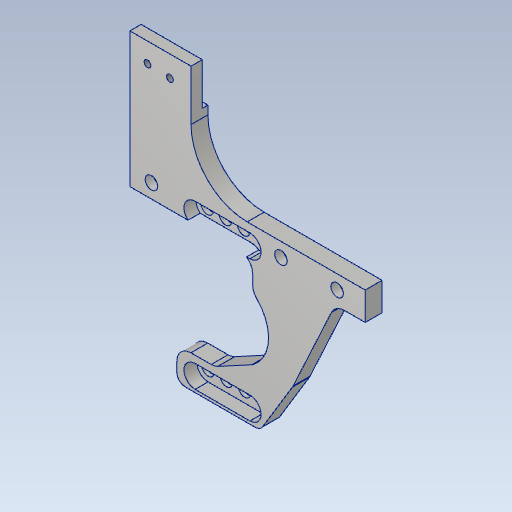
# Autodesk Inventor part: Extruder bracket
Saved by Autodesk Inventor 2020 (Build 240168000, 168)
## iProperties
Created: 2018-10-20
Part Number: Extruder bracket
Material: Aluminum 6061
Document SubType Name: Modeling
Designer: LillaHunden
Density: 2.7 g/cm^3
Appearance: Aluminum - Flat
Mass: 27.8066 g
Surface Area: 65.7368 cm^2
Volume: 10.2987 cm^3
Author: LillaHunden
Autodesk Inventor part; units mm, degrees
sketch "Sketch3" plane through (0, 0, 0) normal (0, 0, 1) x (1, 0, 0)
  line L0 (-29.642335, -32.061774) -> (11.628959, -32.061774)
  line L1 (11.628959, -32.061774) -> (11.628959, 19.831605)
  line L2 (11.628959, 19.831605) -> (37.40227, 19.831605)
  line L3 (37.40227, 19.831605) -> (37.40227, 29.831605)
  line L4 (37.40227, 29.831605) -> (-52.692966, 29.831605)
  line L5 (-52.692966, 29.831605) -> (-52.692966, 19.831605)
  line L6 (-52.692966, 19.831605) -> (-2.658885, 19.831605)
  line L7 (-2.658885, 19.831605) -> (-2.658885, -20.52891)
  line L8 (-2.658885, -20.52891) -> (-29.642335, -20.52891)
  line L9 (-29.642335, -20.52891) -> (-29.642335, -32.061774)
  line L10 (37.40227, 19.831605) -> (-46.39773, 19.831605)
  point P0 (0, 0)
  constraints: 20 end point, 9 perpendicular, 1 horizontal, 1 horizontal alignment, 1 point on line
extrude "Extrusion3" add sketch "Sketch3" along normal blind 6
sketch "Sketch4" plane through (0, 0, 6) normal (0, 0, 1) x (1, 0, 0)
  circle A0 centre (-10.748341, -2.098696) radius 3.15 construction
  circle A1 centre (-10.748341, -2.098696) radius 13.750611
  point P0 (0, 0)
  constraints: 1 centre point, 1 coincident
extrude "Extrusion4" cut sketch "Sketch4" against normal through all
sketch "Sketch5" plane through (0, 0, 0) normal (0, 0, -1) x (-1, 0, 0)
  line L0 (-11.628959, -32.061774) -> (-11.628959, 19.831605)
  line L1 (-11.628959, -12.820332) -> (-26.727339, 19.831605)
  line L2 (-11.628959, 19.831605) -> (-37.40227, 19.831605)
  point P0 (0, 0)
  constraints: 2 end point, 2 point on line
extrude "Extrusion5" add sketch "Sketch5" against normal up to surface (6 mm away)
sketch "Sketch6" plane through (0, 0, 6) normal (0, 0, 1) x (1, 0, 0)
  line L0 (-2.658885, -20.52891) -> (-29.642335, -20.52891)
  line L1 (-2.658885, -13.21805) -> (-2.658885, -20.52891)
  line L2 (-16.15061, -20.52891) -> (-2.658885, -13.21805)
  point P0 (0, 0)
  constraints: 2 end point, 2 midpoint
ref_plane "Work Plane1" through (-29.642335, -32.061774, 0) normal (0, 0, 1) x (1, 0, 0)
extrude "Extrusion6" add sketch "Sketch6" against normal up to surface (6 mm away)
sketch "Sketch7" plane through (0, 0, 0) normal (0, 0, -1) x (-1, 0, 0)
  line L0 (29.642335, -32.061774) -> (-11.628959, -32.061774)
  line L1 (0, -32.061774) -> (-11.628959, -12.820332)
  line L2 (-11.628959, -32.061774) -> (-11.628959, -12.820332)
  point P0 (0, 0)
  constraints: 2 end point, 1 point on line
extrude "Extrusion7" cut sketch "Sketch7" against normal through all
fillet "Fillet1" radius 5 6 edges at (-16.1506, -20.5289, 3) (-2.6589, -13.218, 3) (11.629, -12.8203, 3) (26.7273, 19.8316, 3) (-2.6589, 9.0207, 3) (-2.6589, 19.8316, 3)
fillet "Fillet2" radius 3 1 edges at (-29.6423, -32.0618, 3)
fillet "Fillet3" radius 3 1 edges at (0, -32.0618, 3)
sketch "Sketch8" plane through (0, 0, 0) normal (0, 0, -1) x (-1, 0, 0)
  line L0 (52.59773, 19.831605) -> (-37.40227, 19.831605) construction
  line L1 (-37.40227, 19.831605) -> (-37.40227, 29.831605) construction
  line L2 (52.59773, 29.831605) -> (-37.40227, 29.831605) construction
  line L3 (52.59773, 19.831605) -> (52.59773, 29.831605) construction
  line L4 (-37.40227, 19.831605) -> (-37.40227, 29.831605) construction
  line L5 (-37.40227, 24.831605) -> (52.692966, 24.831605) construction
  line L6 (52.692966, 29.831605) -> (52.692966, 19.831605) construction
  point P0 (0, 0)
  point P1 (-27.40227, 24.831605)
  point P2 (-7.40227, 24.831605)
  point P3 (38.692966, 24.831605)
  dimension "d20" = 10
  dimension "d21" = 14
  dimension "d23" = 20
  constraints: 3 point on line, 2 end point, 2 midpoint
  measures "d20" distance from line of L1 point (-27.402, 24.832)
  measures "d21" distance from line of L6 point (38.693, 24.832)
  measures "d23" distance of point (-7.402, 24.832) point (-27.402, 24.832)
sketch "Sketch9" plane through (0, 0, 0) normal (0, 0, -1) x (-1, 0, 0)
  point P0 (-27.40227, 24.831605)
  point P1 (-7.40227, 24.831605)
  point P2 (38.692966, 24.831605)
hole "Hole1" at (27.40227, 24.831605, 0) at (7.40227, 24.831605, 0) at (-38.692966, 24.831605, 0) direction (0, 0, 1) diameter 4.5 depth 6 counterbore diameter 8.1 counterbore depth 3
sketch "Sketch11" plane through (0, 0, 0) normal (0, 0, -1) x (-1, 0, 0)
  arc A0 (1.642335, 27.938226) -> (-1.357665, 24.938226) centre (1.642335, 24.938226) ccw construction
  line L0 (-1.357665, 12.938226) -> (-1.357665, 24.938226) construction
  line L1 (-1.357665, 12.938226) -> (29.642335, 12.938226) construction
  line L2 (29.642335, 24.938226) -> (29.642335, 12.938226) construction
  arc A1 (29.642335, 24.938226) -> (26.642335, 27.938226) centre (26.642335, 24.938226) ccw construction
  line L3 (1.642335, 27.938226) -> (26.642335, 27.938226) construction
  circle A2 centre (10.142335, 22.938226) radius 2.15
  circle A3 centre (23.142335, 22.938226) radius 2.15
  circle A4 centre (16.642335, 22.938226) radius 2.15
  circle A5 centre (3.642335, 22.938226) radius 2.15
  point P0 (0, 0)
  point P1 (16.642335, 22.938226)
  point P2 (10.142335, 22.938226)
  point P3 (3.642335, 22.938226)
sketch "Sketch12" plane through (0, 0, 6) normal (0, 0, 1) x (1, 0, 0)
  point P0 (-3.642335, -27.061774)
  point P1 (-23.142335, -27.061774)
  point P2 (-16.642335, -27.061774)
  point P3 (-10.142335, -27.061774)
hole "Hole5" at (-3.642335, -27.061774, 6) at (-23.142335, -27.061774, 6) at (-16.642335, -27.061774, 6) at (-10.142335, -27.061774, 6) direction (0, 0, -1) diameter 4.5 depth 6 counterbore diameter 8 counterbore depth 4.6
sketch "Sketch13" plane through (-52.692966, 19.831605, 0) normal (-1, 0, 0) x (0, 0, 1)
  line L0 (0, 10) -> (0, 0) projected
  line L1 (0, 0) -> (6, 0) projected
  line L2 (6, 10) -> (6, 0) projected
  line L3 (0, 10) -> (6, 10) projected
  point P0 (0, -19.831605)
ref_plane "Work Plane2" through (-46.59773, 19.831605, 6) normal (-1, 0, 0) x (0, 0, 1)
extrude "Extrusion8" cut sketch "Sketch13" against normal up to surface (6.095236 mm away)
chamfer "Chamfer2" distance 0.1 angle 45 3 edges at (-38.693, 20.7816, 0) (7.4023, 20.7816, 0) (27.4023, 20.7816, 0)
sketch "Sketch14" plane through (37.40227, 29.831605, 6) normal (0, 1, 0) x (1, 0, 0)
  line L0 (-84, 0) -> (-84, 6)
  line L1 (0, 0) -> (-84, 0)
  line L2 (-84, 6) -> (-62, 6)
  line L3 (-62, 6) -> (-62, 0)
  line L4 (-62, 0) -> (-84, 0)
  line L5 (-84, 0) -> (-84, 6)
  line L6 (-28.762831, -334.839832) -> (-28.762831, 75.160168) construction
  point P0 (-37.40227, 6)
  dimension "d68" = 22
  constraints: 10 end point, 2 parallel, 1 horizontal, 1 perpendicular, 1 point on line
  measures "d68" distance of L0.end L2.end
ref_plane "Work Plane3" through (-348.360561, 52.831605, 2) normal (0, 1, 0) x (0, 0, 1)
extrude "Extrusion9" add sketch "Sketch14" along normal up to surface (23 mm away)
sketch "Sketch15" plane through (-46.59773, 52.831605, 6) normal (0, 1, 0) x (1, 0, 0)
  line L0 (0, 0) -> (22, 0)
  line L1 (22, 0) -> (22, 4)
  line L2 (22, 4) -> (0, 4)
  line L3 (0, 4) -> (0, 0)
  line L4 (0, 6) -> (22, 6) projected
  point P0 (46.59773, 6)
  dimension "d64" = 22
  dimension "d65" = 2
  constraints: 8 end point, 2 parallel, 1 horizontal, 1 perpendicular
  measures "d64" distance between parallel lines of L3 L1
  measures "d65" distance between parallel lines of L4 L2
extrude "Extrusion10" add sketch "Sketch15" along normal blind 15
fillet "Fillet4" radius 20 1 edges at (-24.5977, 29.8316, 3)
sketch "Sketch16" plane through (-24.59773, 52.831605, 2) normal (0, 0, -1) x (-1, 0, 0)
  line L0 (22, 0) -> (22, 15) projected
  line L1 (0, 15) -> (22, 15) projected
  point P0 (-24.59773, -52.831605)
  point P1 (15.5, 8)
  point P2 (7.5, 7.52606)
  dimension "d70" = 6.5
  dimension "d71" = 7
  dimension "d72" = 8
  measures "d70" distance from line of L0 point (15.5, 8)
  measures "d71" distance from line of point (15.5, 8) L1
  measures "d72" horizontal distance of point (15.5, 8) point (7.5, 7.526)
hole "Hole7" at (-40.09773, 60.831605, 2) at (-32.09773, 60.357664, 2) direction (0, 0, 1) diameter 2.459 end through all thread size "M3x0.5" class "6H" standard "ISO Metric profile"
sketch "Sketch18" plane through (0, 0, 6) normal (0, 0, 1) x (1, 0, 0)
  point P0 (-23.142335, 22.938226)
  point P1 (-16.642335, 22.938226)
  point P2 (-10.142335, 22.938226)
  point P3 (-3.642335, 22.938226)
hole "Hole9" at (-23.142335, 22.938226, 6) at (-16.642335, 22.938226, 6) at (-10.142335, 22.938226, 6) at (-3.642335, 22.938226, 6) direction (0, 0, -1) diameter 4.5 depth 6 counterbore diameter 8 counterbore depth 4.3
move faces "Move1" translate (0.25, 0, 0) faces at (-46.59773, 30.831605, 2.666667) (-34.295661, 44.021632, 6)
sketch "Sketch19" plane through (-4.59773, 29.831605, 6) normal (0, 0, 1) x (1, 0, 0)
  circle A0 centre (-18.544605, -6.893378) radius 2.25
  circle A1 centre (0.955395, -6.893378) radius 2.25
  line L0 (-18.544605, -6.893378) -> (0.955395, -6.893378) construction
  line L1 (-18.544605, -10.893378) -> (0.955395, -10.893378)
  line L2 (0.955395, -2.893378) -> (-18.544605, -2.893378)
  arc A2 (-18.544605, -2.893378) -> (-18.544605, -10.893378) centre (-18.544605, -6.893378) ccw
  arc A3 (0.955395, -10.893378) -> (0.955395, -2.893378) centre (0.955395, -6.893378) ccw
  point P0 (4.59773, -29.831605)
  point P1 (-8.794605, -6.893378)
  constraints: 8 end point, 4 point on circle, 4 tangent, 2 centre point, 1 horizontal, 1 midpoint, 1 parallel
extrude "Extrusion11" cut sketch "Sketch19" against normal up to surface (4.3 mm away) contours A0 | A1 | A2 L2 A3 L1
sketch "Sketch20" plane through (-4.59773, 29.831605, 6) normal (0, 0, 1) x (1, 0, 0)
  circle A0 centre (-18.544605, -56.893378) radius 2.25
  circle A1 centre (0.955395, -56.893378) radius 2.25
  line L0 (-18.544605, -56.893378) -> (0.955395, -56.893378) construction
  line L1 (-18.544605, -60.893378) -> (0.955395, -60.893378)
  line L2 (0.955395, -52.893378) -> (-18.544605, -52.893378)
  arc A2 (-18.544605, -52.893378) -> (-18.544605, -60.893378) centre (-18.544605, -56.893378) ccw
  arc A3 (0.955395, -60.893378) -> (0.955395, -52.893378) centre (0.955395, -56.893378) ccw
  point P0 (4.59773, -29.831605)
  point P1 (-8.794605, -56.893378)
  constraints: 8 end point, 4 point on circle, 4 tangent, 2 centre point, 1 horizontal, 1 midpoint, 1 parallel
extrude "Extrusion12" cut sketch "Sketch20" against normal up to surface (4.6 mm away)
fillet "Fillet5" radius 5 1 edges at (-29.6423, -20.5289, 3)
body "Solid2"
